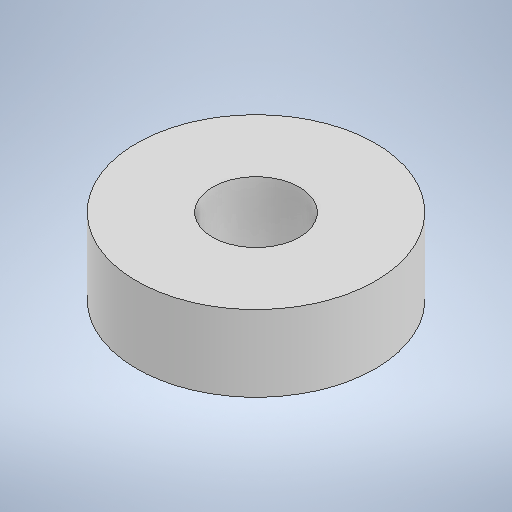
# Autodesk Inventor part: Lager_608ZZ
Saved by Autodesk Inventor 2025 (Build 290162000, 162)
## iProperties
Created: 2026-07-08
Part Number: Lager_608ZZ
Material: Generisch
Document SubType Name: Modeling
Designer: wavid
Mass: 2.30907 g
Surface Area: 13.1947 cm^2
Volume: 2.30907 cm^3
Density: 1 g/cm^3
Appearance: Vorgabe
Author: wavid
Autodesk Inventor part; units mm, degrees
ref_plane "YZ Plane" through (0, 0, 0) normal (1, 0, 0) x (0, 1, 0)
ref_plane "XZ Plane" through (0, 0, 0) normal (0, 1, 0) x (-1, 0, 0)
ref_plane "XY Plane" through (0, 0, 0) normal (0, 0, 1) x (1, 0, 0)
sketch "Skizze1" plane through (0, 0, 0) normal (0, 0, 1) x (1, 0, 0)
  circle A0 centre (0, 0) radius 11
  constraints: 1 centre point
extrude "Extrusion1" add sketch "Skizze1" along normal blind 7
sketch "Skizze2" plane through (0, 0, 0) normal (0, 0, 1) x (1, 0, 0)
  circle A0 centre (0, 0) radius 4
  constraints: 1 centre point
extrude "Extrusion2" cut sketch "Skizze2" along normal blind 7.2
